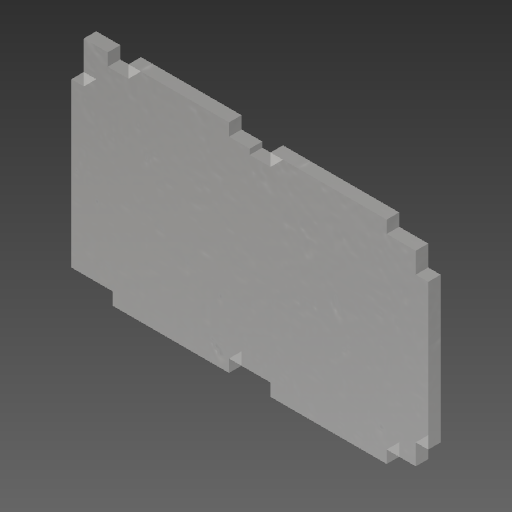
# Autodesk Inventor part: top
Saved by Autodesk Inventor 2019 (Build 230136000, 136)
## iProperties
Created: 2019-05-01
Part Number: top
Material: Acrylic, Clear
Document SubType Name: Modeling
Designer: skylercleland
Density: 1.19 g/cm^3
Appearance: Transparent - Clear
Author: skylercleland
Autodesk Inventor part; units mm, degrees
ref_plane "YZ Plane" through (0, 0, 0) normal (1, 0, 0) x (0, 1, 0)
ref_plane "XZ Plane" through (0, 0, 0) normal (0, 1, 0) x (-1, 0, 0)
ref_plane "XY Plane" through (0, 0, 0) normal (0, 0, 1) x (1, 0, 0)
sketch "Sketch1" plane through (0, 0, 0) normal (0, 0, 1) x (1, 0, 0)
  line L0 (0, -46.3) -> (0, 3) projected
  line L1 (3, 3) -> (43, 3) projected
  line L2 (3, 3) -> (0, 3) projected
  line L3 (43, 0) -> (43, 3) projected
  line L4 (43, 1.7) -> (86, 1.7) projected
  line L5 (86, -1.3) -> (86, 1.7) projected
  line L6 (86, -1.3) -> (86, -46.3) projected
  line L7 (86, -46.3) -> (86, -49.3) projected
  line L8 (86, -49.3) -> (0, -49.3) projected
  line L9 (0, -46.3) -> (0, -49.3) projected
  line L10 (3, -46.3) -> (0, -46.3) projected
  line L11 (3, 3) -> (3, 0) projected
  line L12 (43, -1.3) -> (43, 1.7) projected
  line L13 (83, -46.3) -> (83, -1.3) projected
  line L14 (83, -46.3) -> (86, -46.3) projected
  line L15 (86, -1.3) -> (86, -46.3) projected
  line L16 (83, -1.3) -> (86, -1.3) projected
  line L17 (83, -46.3) -> (76, -46.3)
  line L18 (76, -46.3) -> (76, -49.3)
  line L19 (83, -1.3) -> (76, -1.3)
  line L20 (76, -1.3) -> (76, 1.7)
  line L21 (43, -1.3) -> (48, -1.3)
  line L22 (48, -1.3) -> (48, 1.7)
  line L23 (43, 0) -> (38, 0)
  line L24 (38, 0) -> (38, 3)
  line L25 (3, -46.3) -> (10, -46.3)
  line L26 (10, -46.3) -> (10, -49.3)
  line L27 (3, 0) -> (3, -7)
  line L28 (3, -7) -> (0, -7)
  line L29 (13.777, 0) -> (8.777, 0)
  line L30 (8.777, 0) -> (8.777, 3)
  line L31 (8.777, 3) -> (13.777, 3)
  line L32 (13.777, 3) -> (13.777, 0)
  line L33 (48, -49.3) -> (38, -49.3)
  line L34 (38, -49.3) -> (38, -46.3)
  line L35 (38, -46.3) -> (48, -46.3)
  line L36 (48, -46.3) -> (48, -49.3)
  line L37 (86, -6.3) -> (83, -6.3)
  line L38 (83, -41.3) -> (86, -41.3)
  point P0 (0, 0)
  point P1 (43, -49.3)
  dimension "d0" = 10
  dimension "d1" = 10
  dimension "d2" = 10
  dimension "d3" = 10
  dimension "d4" = 10
  dimension "d5" = 5
  dimension "d6" = 5
  dimension "d7" = 5
  dimension "d10" = 5
  dimension "d11" = 5
  constraints: 44 end point, 12 point on line, 10 perpendicular, 7 horizontal, 4 parallel, 2 horizontal alignment, 2 midpoint, 1 vertical
  measures "d0" distance between parallel lines of L5 L20
  measures "d1" distance between parallel lines of L7 L18
  measures "d2" distance between parallel lines of L9 L26
  measures "d3" distance between parallel lines of L36 L34
  measures "d4" distance between parallel lines of L2 L28
  measures "d5" distance between parallel lines of L32 L30
  measures "d6" distance between parallel lines of L3 L24
  measures "d7" distance between parallel lines of L12 L22
  measures "d10" distance between parallel lines of L16 L37
  measures "d11" distance between parallel lines of L38 L14
extrude "Extrusion1" add sketch "Sketch1" along normal blind 3 contours L0 L28 L27 L11 L1 L30 L29 L32 L24 L23 L12 L21 L22 L4 L20 L19 L13 L17 L18 L8 L36 L35 L34 L26 L25 L10 | L38 L13 L37 L6
body "Solid1"
